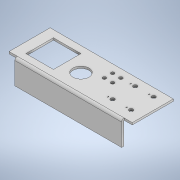
# Autodesk Inventor part: Labview Training Faceplate
Saved by Autodesk Inventor 2021.3 (Build 253353010, 353A)
## iProperties
Created: 2022-07-29
Part Number: Labview Training Faceplate
Material: Generic
Document SubType Name: Modeling
Designer: dheard
Density: 1 g/cm^3
Appearance: Default
Author: dheard
Autodesk Inventor part; units mm, degrees
ref_plane "YZ Plane" through (0, 0, 0) normal (1, 0, 0) x (0, 1, 0)
ref_plane "XZ Plane" through (0, 0, 0) normal (0, 1, 0) x (-1, 0, 0)
ref_plane "XY Plane" through (0, 0, 0) normal (0, 0, 1) x (1, 0, 0)
sketch "Sketch1" plane through (0, 0, 0) normal (0, 1, 0) x (-1, 0, 0)
  line L0 (150, -50) -> (-150, -50)
  line L1 (-150, -50) -> (-150, 50)
  line L2 (150, 50) -> (150, -50)
  line L3 (-130, 50) -> (-130, 105)
  line L4 (-130, 105) -> (130, 105)
  line L5 (130, 105) -> (130, 50)
  line L6 (-150, 50) -> (-130, 50)
  line L7 (130, 50) -> (150, 50)
  point P0 (0, 0)
  dimension "d0" = 100
  dimension "d1" = 55
  dimension "d2" = 300
  dimension "d3" = 20
  dimension "d4" = 20
  dimension "d5" = 150
  dimension "d6" = 50
  constraints: 16 end point, 4 parallel, 2 horizontal alignment, 1 horizontal, 1 perpendicular
  measures "d0" distance between parallel lines of L7 L0
  measures "d1" distance between parallel lines of L4 L7
  measures "d2" distance between parallel lines of L1 L2
  measures "d3" distance between parallel lines of L5 L2
  measures "d4" distance between parallel lines of L1 L3
  measures "d5" distance from line of point (0, 0) L1
  measures "d6" distance from line of point (0, 0) L0
extrude "Extrusion1" add sketch "Sketch1" along normal blind 5
sketch "Sketch3" plane through (0, 5, 0) normal (0, 1, 0) x (1, 0, 0)
  line L0 (-125, 33) -> (-58, 33)
  line L1 (-58, 33) -> (-58, -34)
  line L2 (-58, -34) -> (-125, -34)
  line L3 (-125, -34) -> (-125, 33)
  line L4 (150, 50) -> (-150, 50) projected
  line L5 (-150, 50) -> (-150, -50) projected
  circle A0 centre (-18, -7) radius 19.5
  line L6 (-34, 9) -> (-2, 9) construction
  line L7 (-2, 9) -> (-2, -23) construction
  line L8 (-2, -23) -> (-34, -23) construction
  line L9 (-34, -23) -> (-34, 9) construction
  circle A1 centre (-34, 9) radius 1.5
  circle A2 centre (-2, -23) radius 1.5
  circle A3 centre (-34, -23) radius 1.5
  circle A4 centre (-2, 9) radius 1.5
  circle A5 centre (77, -25) radius 4.75
  circle A6 centre (77, 30) radius 4.75
  circle A7 centre (122, -25) radius 4.75
  circle A8 centre (122, 30) radius 4.75
  circle A9 centre (22, 10) radius 4.15
  circle A10 centre (42, 10) radius 4.15
  circle A11 centre (42, 30) radius 4.15
  circle A12 centre (22, 30) radius 4.15
  line L10 (66, 31.3) -> (66, 28.7) construction
  line L11 (66.65, 31.3) -> (66.65, 28.7)
  line L12 (65.35, 28.7) -> (65.35, 31.3)
  arc A13 (66.65, 31.3) -> (65.35, 31.3) centre (66, 31.3) ccw
  arc A14 (65.35, 28.7) -> (66.65, 28.7) centre (66, 28.7) ccw
  line L13 (66, -23.7) -> (66, -26.3) construction
  line L14 (66.65, -23.7) -> (66.65, -26.3)
  line L15 (65.35, -26.3) -> (65.35, -23.7)
  arc A15 (66.65, -23.7) -> (65.35, -23.7) centre (66, -23.7) ccw
  arc A16 (65.35, -26.3) -> (66.65, -26.3) centre (66, -26.3) ccw
  line L16 (110.35, -26.3) -> (110.35, -23.7)
  line L17 (111, -23.7) -> (111, -26.3) construction
  line L18 (111.65, -23.7) -> (111.65, -26.3)
  arc A17 (111.65, -23.7) -> (110.35, -23.7) centre (111, -23.7) ccw
  arc A18 (110.35, -26.3) -> (111.65, -26.3) centre (111, -26.3) ccw
  line L19 (110.35, 28.7) -> (110.35, 31.3)
  line L20 (111, 31.3) -> (111, 28.7) construction
  line L21 (111.65, 31.3) -> (111.65, 28.7)
  arc A19 (111.65, 31.3) -> (110.35, 31.3) centre (111, 31.3) ccw
  arc A20 (110.35, 28.7) -> (111.65, 28.7) centre (111, 28.7) ccw
  point P0 (66, 30)
  point P1 (66, -25)
  point P2 (111, -25)
  point P3 (111, 30)
  dimension "d11" = 67
  dimension "d12" = 67
  dimension "d13" = 17
  dimension "d15" = 25
  dimension "d16" = 39
  dimension "d17" = 40
  dimension "d18" = 40
  dimension "d19" = 32
  dimension "d20" = 32
  dimension "d23" = 16
  dimension "d24" = 16
  dimension "d25" = 3
  dimension "d26" = 3
  dimension "d27" = 3
  dimension "d28" = 3
  dimension "d29" = 9.5
  dimension "d30" = 45
  dimension "d31" = 55
  dimension "d32" = 20
  dimension "d34" = 8.3
  dimension "d36" = 20
  dimension "d37" = 20
  dimension "d38" = 20
  dimension "d39" = 40
  dimension "d40" = 35
  dimension "d41" = 11
  dimension "d42" = 2.6
  dimension "d43" = 1.3
  dimension "d44" = 2.6
  dimension "d45" = 1.3
  dimension "d46" = 2.6
  dimension "d47" = 1.3
  dimension "d48" = 2.6
  dimension "d49" = 1.3
  dimension "d50" = 11
  constraints: 48 end point, 21 centre point, 16 point on circle, 16 tangent, 8 horizontal alignment, 8 parallel, 6 equal radius, 6 vertical alignment, 4 coincident, 4 midpoint, 4 vertical, 2 horizontal, 2 perpendicular
  measures "d11" distance between parallel lines of L1 L3
  measures "d12" distance between parallel lines of L2 L0
  measures "d13" distance between parallel lines of L4 L0
  measures "d15" distance between parallel lines of L5 L3
  measures "d16" diameter of A0
  measures "d17" distance from line of L0 A0.centre
  measures "d18" distance from line of A0.centre L1
  measures "d19" distance between parallel lines of L7 L9
  measures "d20" distance between parallel lines of L6 L8
  measures "d23" distance from line of A0.centre L6
  measures "d24" distance from line of A0.centre L9
  measures "d25" diameter of A1
  measures "d26" diameter of A4
  measures "d27" diameter of A2
  measures "d28" diameter of A3
  measures "d29" diameter of A5
  measures "d30" distance of A8.centre A6.centre
  measures "d31" distance of A7.centre A8.centre
  measures "d32" distance from line of L4 A6.centre
  measures "d34" diameter of A9
  measures "d36" distance of A10.centre A9.centre
  measures "d37" distance of A10.centre A11.centre
  measures "d38" distance from line of L4 A12.centre
  measures "d39" horizontal distance of A0.centre A12.centre
  measures "d40" distance of A11.centre A6.centre
  measures "d41" distance of A6.centre point (66, 30)
  measures "d42" distance of L10.start L10.end
  measures "d43" distance between parallel lines of L11 L12
  measures "d44" distance of L13.start L13.end
  measures "d45" distance between parallel lines of L14 L15
  measures "d46" distance of L17.start L17.end
  measures "d47" distance between parallel lines of L18 L16
  measures "d48" distance of L20.start L20.end
  measures "d49" distance between parallel lines of L21 L19
  measures "d50" distance of A8.centre point (111, 30)
extrude "Extrusion2" cut sketch "Sketch3" against normal through all contours L0 L1 L2 L3 | A0 | A5 | A6 | A7 | A8 | A9 | A10 | A11 | A12 | L11 A14 L12 A13 | L14 A16 L15 A15 | L16 A17 L18 A18 | L19 A19 L21 A20
sketch "Sketch2" plane through (0, 0, 0) normal (0, 1, 0) x (1, 0, 0)
  line L0 (-144.7476, -50) -> (134.453, -50)
  point P0 (0, 0)
  point P1 (-130, -50)
  point P2 (130, -50)
  constraints: 2 end point, 2 horizontal alignment
bend part "Bend Part2" radius 1 angle 90 line through (-144.7476, 0, 50) along (1, 0, 0) centre toward (0, -1, 0) moving side (0, 0, 1) both sides no
equation "\"d5\" = 0.5 * d2"
equation "\"d6\" = 0.5 * d0"
equation "\"d23\" = 0.5 * d20"
equation "\"d24\" = 0.5 * d19"
body "Solid1"
